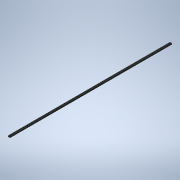
# Autodesk Inventor part: SSE2B-MX13-970_r
Saved by Autodesk Inventor 2021 (Build 250183000, 183)
## iProperties
Created: 2025-02-22
Part Number: SSE2B-MX13-970_r
Material: Generic
Catalog Web Link: www.cadenas.de
Description: SSEB, SSEB-MX, SSEBV, SSEBV-MX, SSE2B, SSE2B-MX, SSE2BV, SSE2BV-MX, SSEBL, SSEBL-MX, SSEBLV, SSEBLV-MX, SSE2BL, SSE2BL-MX, SSE2BLV, SSE2BLV-MX, SEB, SEBV, SE2B, SE2BV, SEBL, SEBLV, SE2BL, SE2BLV_rail-Miniature Linear Guides - Short Block, Standard Preload - High/Precision Grade
Vendor: MISUMI
Document SubType Name: Modeling
Designer: psAdmin
Manufacturer: MISUMI
Mass: 75.3938 g
Surface Area: 469.133 cm^2
Volume: 75.3938 cm^3
Density: 1 g/cm^3
Appearance: PSOLRGB-175-175-175
Category: PARTsolutions
Company: MISUMI
Title: SSE2B-MX13-970
Author: Cadenas PARTsolutions
Comments: Miniature Linear Guides - Short Block, Standard Preload - High/Precision Grade
PSOL_IDENT_0: {$CADENAS_DATA/23d-libs/misumi/metric/06_linear_guides/seb_series/seb_rail.prj},403 {VTYP=3D},{NB=SS
PSOL_IDENT_1: E2B-MX13-970_r},{LINA=SSE2B-MX13-970},{NN=SSEB, SSEB-MX, SSEBV, SSEBV-MX, SSE2B, SSE2B-MX, SSE2BV, S
PSOL_IDENT_2: SE2BV-MX, SSEBL, SSEBL-MX, SSEBLV, SSEBLV-MX, SSE2BL, SSE2BL-MX, SSE2BLV, SSE2BLV-MX, SEB, SEBV, SE2
PSOL_IDENT_3: B, SE2BV, SEBL, SEBLV, SE2BL, SE2BLV_rail},{DATE=17.02.2022 00:32:34},{GEOMDATE=21.01.2022 00:02:30}
PSOL_IDENT_4: ,{VERSION=},{LINEID=230},{WBVAR=TS,ST,MAT,MX,NOB,LT,LS,ALT1,ALT2,ALT4},{WBNUMERIC=LS}  {NB=SSE2B-MX1
PSOL_IDENT_5: 3-970_r},{LINA=SSE2B-MX13-970},{KT=DUMMY},{PN=SSE2B-MX13-970},{RT=B},{TS=},{TS1=  '','Advanced','V','
PSOL_IDENT_6: Precision'  },{TYPE=SSE2B},{ST=S},{MAT=S},{MX=-MX},{MXALG='', 'w/o MX(Lubrication unit)', '-MX', 'wi
PSOL_IDENT_7: th MX(Lubrication unit)'},{NOB=2},{H=13},{LT=Selectable},{LTALG='Selectable','Selectable','Configura
PSOL_IDENT_8: ble','Configurable'},{LS=970},{W=27},{L1=33.9},{B=20},{C=15},{S=M3x3.5},{L2=19.9},{K=10.0},{CBB=0.5}
PSOL_IDENT_9: ,{W1=12},{W2=7.5},{H1=7.5},{CAA=0.5},{DD1DD2HH=3.5x6x4.5},{F=25},{G=10.0},{DD1=3.500},{DD2=6.000},{H
PSOL_IDENT_10: H=4.500},{ALT1=},{ALT1ALG='', 'Not applicable'},{MC=M4},{MC1=4.0},{ALT2=},{ALT2L=5.0},{ALT2N=5},{M=3
PSOL_IDENT_11: 9},{LL=},{L0=95,120,145,170,195,220,245,270,295,320,345,370,395,420,445,470,495,520,545,570,595,620,
PSOL_IDENT_12: 645,670,695,720,745,770,795,820,845,870,895,920,945,970},{REC1=   '','w/o Rail Ends Cut alteration','
PSOL_IDENT_13: -LLC','with LLC (Left End Cut)','-RLC','with RLC (Right End Cut)','-LLC-RLC','with Both End Cut'   }
PSOL_IDENT_14: ,{ST1='S', 'w/o Surface Treatment','R','Low Temperature Black Chrome Plating'},{MAT2= 'S','Stainless
PSOL_IDENT_15: Steel','','Carbon Steel' },{NL=242.500},{ALT4=},{ALT4ALG= '','N/A' },{CA1=0.3},{CA2=0.5},{VA1=2.3},
PSOL_IDENT_16: {HA1=2.0},{HA2=12.5830},{WA1=2.5298},{WA2=1.0},{RA1=2.64},{POIA1=0.1820},{NA1=38},{LSC=0.0},{MS=0.0}
NB: SSE2B-MX13-970_r
NN: SSEB, SSEB-MX, SSEBV, SSEBV-MX, SSE2B, SSE2B-MX, SSE2BV, SSE2BV-MX, SSEBL, SSEBL-MX, SSEBLV, SSEBLV-MX, SSE2BL, SSE2BL-MX, SSE2BLV, SSE2BLV-MX, SEB, SEBV, SE2B, SE2BV, SEBL, SEBLV, SE2BL, SE2BLV_rail
NT: Miniature Linear Guides - Short Block, Standard Preload - High/Precision Grade
NBSYN: $PN._r
LINA: SSE2B-MX13-970
CATALOG: Misumi
PN: SSE2B-MX13-970
TS: Advanced
ST: w/o Surface Treatment
MAT: Stainless Steel
MX: with MX(Lubrication unit)
NOB: 2
H: 13
LT: Selectable
LS: 970
W: 27
L1: 33.9
B: 20
C: 15
S: M3x3.5
L2: 19.9
K: 10
CBB: 0.5
W1: 12
W2: 7.5
H1: 7.5
CAA: 0.5
DD1DD2HH: 3.5x6x4.5
F: 25
G: 10
ALT1: Not applicable
ALT2: w/o Rail Ends Cut alteration
ALT4: N/A
NA1: 38
SUPPLIER: MISUMI
ARTICLENO: SSE2B-MX13-970_r
BOMINFO: SSE2B-MX13-970
CREATOR: CADENAS GmbH
Autodesk Inventor part; units mm, degrees
sketch "Sketch_12" plane through (0, 0, 0) normal (0, 0, 1) x (1, 0, 0)
  line L0 (-6, 7.2) -> (-6, 6.4649)
  line L1 (-6, 6.4649) -> (-5.6315, 6.2522)
  arc A0 (-5.1112, 5.7) -> (-5.6315, 6.2522) centre (-6.2915, 5.109) ccw
  line L2 (-5.1112, 5.7) -> (-4, 5.7)
  line L3 (-4, 5.7) -> (-4, 4.7)
  line L4 (-4, 4.7) -> (-5.1112, 4.7)
  arc A1 (-5.6315, 4.1478) -> (-5.1112, 4.7) centre (-6.2915, 5.291) ccw
  line L5 (-5.6315, 4.1478) -> (-6, 3.9351)
  line L6 (-6, 3.9351) -> (-6, 0.5)
  line L7 (-6, 0.5) -> (-5.5, 0)
  line L8 (-5.5, 0) -> (5.5, 0)
  line L9 (5.5, 0) -> (6, 0.5)
  line L10 (6, 0.5) -> (6, 3.9351)
  line L11 (6, 3.9351) -> (5.6315, 4.1478)
  arc A2 (5.1112, 4.7) -> (5.6315, 4.1478) centre (6.2915, 5.291) ccw
  line L12 (5.1112, 4.7) -> (4, 4.7)
  line L13 (4, 4.7) -> (4, 5.7)
  line L14 (4, 5.7) -> (5.1112, 5.7)
  arc A3 (5.6315, 6.2522) -> (5.1112, 5.7) centre (6.2915, 5.109) ccw
  line L15 (5.6315, 6.2522) -> (6, 6.4649)
  line L16 (6, 6.4649) -> (6, 7.2)
  line L17 (6, 7.2) -> (5.7, 7.5)
  line L18 (5.7, 7.5) -> (-5.7, 7.5)
  line L19 (-5.7, 7.5) -> (-6, 7.2)
  constraints: 40 end point, 8 point on circle, 4 centre point
extrude "Extrusion1" add sketch "Sketch_12" along normal mid plane 970
sketch "Sketch2" plane through (-5.7, 7.5, 485) normal (0, 1, 0) x (1, 0, 0)
  point P0 (5.7, 960)
hole "Hole1" at (0, 7.5, -475) direction (0, -1, 0) diameter 3.5 depth 7.5 counterbore diameter 6 counterbore depth 4.5
pattern_linear "Rectangular Pattern1" count 39 spacing 25 along (0, 0, 1) of "Hole1"
ref_plane "rail_to_adjusting_block_XY" through (0, 0, -475) normal (0, 1, 0) x (1, 0, 0)
ref_plane "rail_to_adjusting_block_YZ" through (0, 0, -475) normal (1, 0, 0) x (0, 0, -1)
ref_plane "rail_to_adjusting_block_ZX" through (0, 0, -475) normal (0, 0, -1) x (0, 1, 0)
ref_plane "to_block_XY" through (0, 7.5, 242.5) normal (0, 0, 1) x (1, 0, 0)
ref_plane "to_block_YZ" through (0, 7.5, 242.5) normal (1, 0, 0) x (0, 1, 0)
ref_plane "to_block_ZX" through (0, 7.5, 242.5) normal (0, 1, 0) x (0, 0, 1)
ref_plane "to_block_2_XY" through (0, 7.5, -242.5) normal (0, 0, 1) x (1, 0, 0)
ref_plane "to_block_2_YZ" through (0, 7.5, -242.5) normal (1, 0, 0) x (0, 1, 0)
ref_plane "to_block_2_ZX" through (0, 7.5, -242.5) normal (0, 1, 0) x (0, 0, 1)
ref_plane "to_kue_XY" through (0, 0, 0) normal (0, 1, 0) x (1, 0, 0)
ref_plane "to_kue_YZ" through (0, 0, 0) normal (1, 0, 0) x (0, 0, -1)
ref_plane "to_kue_ZX" through (0, 0, 0) normal (0, 0, -1) x (0, 1, 0)
body "Solid1"
